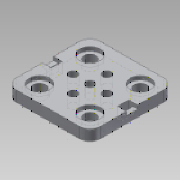
# Autodesk Inventor part: Micro V Plate
Saved by Autodesk Inventor 2013 SP2 (Build 170200200, 200)
## iProperties
IsCustomPart: 0
Created: 2013-06-20
Part Number: Micro V Plate
Material: Aluminum 6061
Document SubType Name: Modeling
Designer: Jon Hollander
Language: en-US
Size Designation: Micro V Plate
Categories: <MemberInstance><Categories><Category DisplayName="Other Parts" InternalName="5aa15e00-363f-49f2-933f-16f664388e3f" Mnemonic="OTHER"><Category DisplayName="Plates" InternalName="59c67330-93a2-418f-82cd-11a50f680607" Mnemonic="PLATES"/></Category><Category DisplayName="DataType" InternalName="23b78d0f-2648-40c6-8793-ca6db495c9e8" Mnemonic="DATATYPE"><CategoryParameter DisplayName="DisplayName" InternalName="05415f3d-3907-474b-a020-eb9d644f4cf3" Mnemonic="DISPLAYNAME"/><CategoryParameter DisplayName="InternalName" InternalName="cf1d0246-76d9-4b4a-8305-fa0409afb5c1" Mnemonic="INTERNALNAME"/><CategoryParameter DisplayName="Folder Name" InternalName="3f06958e-8713-4116-9be7-ed6184ecc97b" Mnemonic="FOLDERNAME"/><CategoryParameter DisplayName="Family Version" InternalName="914462f6-6e19-4b14-ba84-155b9680b1d0" Mnemonic="FAMILYREVISION"/><CategoryParameter DisplayName="ClipFormat" InternalName="bc51e27b-3422-4e78-93ef-cec197ddf230" Mnemonic="CLIPFORMAT"/><CategoryParameter DisplayName="IsMetric" InternalName="e2385c5b-1ea4-4823-96a8-8de651266ec3" Mnemonic="ISMETRIC"/><CategoryParameter DisplayName="Description" InternalName="13903e3d-64b1-4950-80da-f627842ea37f" Mnemonic="DESCRIPTION"/><CategoryParameter DisplayName="StdsOrg" InternalName="8f5914e1-4693-403f-8ab5-d37768198c9d" Mnemonic="STDSORG"/><CategoryParameter DisplayName="Standard" InternalName="0c0a119c-1e12-4c84-803f-101930972f5e" Mnemonic="STANDARD"/><CategoryParameter DisplayName="Manufacturer" InternalName="cd6c7a72-a28a-4e50-99a9-2c7f4e13e5ad" Mnemonic="MANUFACTURER"/><CategoryParameter DisplayName="Member Revision" InternalName="a65d44b9-392f-4f4f-857b-e4b3d54996fe" Mnemonic="MEMBERREVISION"/><CategoryParameter DisplayName="Standard Revision" InternalName="91d5a463-65c2-4fde-b823-3b7fea5e8e17" Mnemonic="STANDARDREVISION"/><CategoryParameter DisplayName="Revision Guid" InternalName="45a75005-10b1-4dfc-8d6d-dfe629f0b93c" Mnemonic="REVISIONGUID"/><CategoryParameter DisplayName="Designation" InternalName="2675968c-4ce5-49e0-a4f5-552d29089031" Mnemonic="DESIGNATION"/><CategoryParameter DisplayName="FileName" InternalName="8b46a4cc-9585-4fed-90c3-899f57e09a73" Mnemonic="FILENAME"/><CategoryParameter DisplayName="Default Row" InternalName="2af9ec52-faaa-4026-b378-f9fa4afca842" Mnemonic="DEFAULTROW"/><Category DisplayName="Part" InternalName="c0e0b642-3bcb-4cc8-9e80-f96d35c4afa4" Mnemonic="PART"><CategoryParameter DisplayName="Material" InternalName="818a152a-d3c3-49ca-80ee-df7d91421b8e" Mnemonic="MATERIAL"/><CategoryParameter DisplayName="Material Key" InternalName="5c9a8adb-dd2b-4535-b97f-0a94a95fe41f" Mnemonic="MATERIALKEY"/><CategoryParameter DisplayName="Part Number" InternalName="016b6077-bfbe-49bd-92c9-d8d59c39c941" Mnemonic="PARTNUMBER"/><CategoryParameter DisplayName="Stock Number" InternalName="4dba7c1c-e26c-444e-836c-b08b433409a8" Mnemonic="STOCKNUMBER"/></Category></Category></Categories><FamilyTemplate Id="Micro V Plate"><FamilyTemplateParameters><FamilyTemplateParameter ObjectType="kPartComponentDefinitionObject" ValueType="xs:string" Id="11" SubObjectId="Material"/><FamilyTemplateParameter ObjectType="kPropertyObject" ValueType="xs:string" Id="19" ObjectReferenceKey="{32853F0F-3444-11d1-9E93-0060B03C1CA6}" SubObjectId="5"/><FamilyTemplateParameter ObjectType="kPropertyObject" ValueType="xs:string" Id="20" ObjectReferenceKey="{32853F0F-3444-11d1-9E93-0060B03C1CA6}" SubObjectId="52"/></FamilyTemplateParameters></FamilyTemplate><CategoryParameterMap><ParamToTemplateMap><ParamToTemplate CategoryParameter="//CategoryParameter[@InternalName='cf1d0246-76d9-4b4a-8305-fa0409afb5c1']" ConstantValue="c0ed0d7d-6565-4805-8c82-f5f5bedef9ef"/><ParamToTemplate CategoryParameter="//CategoryParameter[@InternalName='45a75005-10b1-4dfc-8d6d-dfe629f0b93c']" ConstantValue="dbef3a4f-6e90-4593-8616-ded3e929c80e"/><ParamToTemplate CategoryParameter="//CategoryParameter[@InternalName='3f06958e-8713-4116-9be7-ed6184ecc97b']" ConstantValue="Micro V Plate"/><ParamToTemplate CategoryParameter="//CategoryParameter[@InternalName='8f5914e1-4693-403f-8ab5-d37768198c9d']" TemplateParameter="5"/><ParamToTemplate CategoryParameter="//CategoryParameter[@InternalName='0c0a119c-1e12-4c84-803f-101930972f5e']" TemplateParameter="6"/><ParamToTemplate CategoryParameter="//CategoryParameter[@InternalName='91d5a463-65c2-4fde-b823-3b7fea5e8e17']" TemplateParameter="7"/><ParamToTemplate CategoryParameter="//CategoryParameter[@InternalName='cd6c7a72-a28a-4e50-99a9-2c7f4e13e5ad']" TemplateParameter="8"/><ParamToTemplate CategoryParameter="//CategoryParameter[@InternalName='13903e3d-64b1-4950-80da-f627842ea37f']" TemplateParameter="10"/><ParamToTemplate CategoryParameter="//CategoryParameter[@InternalName='05415f3d-3907-474b-a020-eb9d644f4cf3']" ConstantValue="Micro V Plate"/><ParamToTemplate CategoryParameter="//CategoryParameter[@InternalName='914462f6-6e19-4b14-ba84-155b9680b1d0']" ConstantValue="11"/><ParamToTemplate CategoryParameter="//CategoryParameter[@InternalName='bc51e27b-3422-4e78-93ef-cec197ddf230']" ConstantValue="CF_INVENTOR.STDPARTS"/><ParamToTemplate CategoryParameter="//CategoryParameter[@InternalName='e2385c5b-1ea4-4823-96a8-8de651266ec3']" ConstantValue="true"/><ParamToTemplate CategoryParameter="//CategoryParameter[@InternalName='2af9ec52-faaa-4026-b378-f9fa4afca842']" ConstantValue="1"/><ParamToTemplate CategoryParameter="//CategoryParameter[@InternalName='8b46a4cc-9585-4fed-90c3-899f57e09a73']" ConstantValue="Micro V Plate"/><ParamToTemplate CategoryParameter="//CategoryParameter[@InternalName='a65d44b9-392f-4f4f-857b-e4b3d54996fe']" ConstantValue="f0f53da8-0783-4aef-9824-e74bb68f6a2c"/><ParamToTemplate CategoryParameter="//CategoryParameter[@InternalName='a65d44b9-392f-4f4f-857b-e4b3d54996fe']" ConstantValue="f0f53da8-0783-4aef-9824-e74bb68f6a2c"/><ParamToTemplate CategoryParameter="//CategoryParameter[@InternalName='2675968c-4ce5-49e0-a4f5-552d29089031']" TemplateParameter="20"/><ParamToTemplate CategoryParameter="//CategoryParameter[@InternalName='818a152a-d3c3-49ca-80ee-df7d91421b8e']" TemplateParameter="11"/><ParamToTemplate CategoryParameter="//CategoryParameter[@InternalName='016b6077-bfbe-49bd-92c9-d8d59c39c941']" TemplateParameter="19"/></ParamToTemplateMap></CategoryParameterMap></MemberInstance>
Mass: 35.4792 g
Surface Area: 69.5498 cm^2
Volume: 13.092 cm^3
Density: 2.71 g/cm^3
Author: Jon Hollander
Autodesk Inventor part; units mm, degrees
ref_plane "Work Plane1" through (0, -18.83, 0) normal (-1, 0, 0) x (0, 0, 1)
ref_plane "YZ Plane" through (0, 0, 0) normal (1, 0, 0) x (0, 1, 0)
ref_plane "XZ Plane" through (0, 0, 0) normal (0, 1, 0) x (-1, 0, 0)
sketch "Sketch1" plane through (0, 0, 0) normal (0, 0, 1) x (1, 0, 0)
  line L0 (-25, -25) -> (25, -25)
  line L1 (25, -25) -> (25, 25)
  line L2 (25, 25) -> (-25, 25)
  line L3 (-25, 25) -> (-25, -25)
  line L4 (-25, -25) -> (25, 25) construction
  line L5 (25, -25) -> (-25, 25) construction
  point P0 (0, 0)
  dimension "Width" = 50
  dimension "Height" = 50
  constraints: 12 end point, 2 midpoint, 2 parallel, 1 horizontal, 1 perpendicular
  measures "Width" distance of L2.end L1.end
  measures "Height" distance of L0.end L1.end
extrude "Extrusion1" add sketch "Sketch1" along normal blind 6.35
sketch "Sketch2" plane through (0, 0, 6.35) normal (0, 0, 1) x (1, 0, 0)
  line L0 (-25, -25) -> (25, -25) projected
  line L1 (25, -25) -> (25, 25) projected
  line L2 (25, 25) -> (-25, 25) projected
  line L3 (-25, 25) -> (-25, -25) projected
  line L4 (0, 25) -> (0, -25) construction
  line L5 (-25, 0) -> (25, 0) construction
  point P0 (0, 0)
  point P1 (0, 0)
  point P2 (-10, 0)
  point P3 (0, 10)
  point P4 (0, -10)
  point P5 (10, 0)
  dimension "d4" = 10
  dimension "d5" = 10
  dimension "d6" = 10
  dimension "d7" = 10
  constraints: 4 end point, 4 midpoint, 4 point on line, 1 coincident
  measures "d4" distance of point (0, 0) point (-10, 0)
  measures "d5" distance of point (10, 0) point (0, 0)
  measures "d6" distance of point (0, 10) point (0, 0)
  measures "d7" distance of point (0, -10) point (0, 0)
hole "Hole1" at (0, 0, 6.35) at (-10, 0, 6.35) at (0, 10, 6.35) at (0, -10, 6.35) at (10, 0, 6.35) direction (0, 0, -1) diameter 5.02 end through all
sketch "Sketch3" plane through (0, 0, 6.35) normal (0, 0, 1) x (1, 0, 0)
  line L0 (-25, -25) -> (25, -25) projected
  line L1 (25, -25) -> (25, 25) projected
  line L2 (25, 25) -> (-25, 25) projected
  line L3 (-25, 25) -> (-25, -25) projected
  line L4 (0, 25) -> (0, -25) construction
  line L5 (25, 0) -> (-25, 0) construction
  line L6 (15, 25) -> (15, -25) construction
  line L7 (-25, -15) -> (25, -15) construction
  point P0 (15, 15)
  point P1 (-15, 15)
  dimension "d15" = 15
  dimension "d16" = 15
  constraints: 8 end point, 4 midpoint, 4 point on line, 2 perpendicular
  measures "d15" distance between parallel lines of L6 L4
  measures "d16" distance between parallel lines of L5 L7
hole "Hole2" at (-15, 15, 6.35) at (15, 15, 6.35) direction (0, 0, -1) diameter 7.14 end through all counterbore diameter 12 counterbore depth 2.18
sketch "Sketch6" plane through (0, 0, 6.35) normal (0, 0, 1) x (1, 0, 0)
  circle A0 centre (-15, 15) radius 6 projected
  circle A1 centre (15, 15) radius 6 projected
  circle A2 centre (0, -10) radius 2.51 projected
  circle A3 centre (-10, 0) radius 2.51 projected
  circle A4 centre (0, 0) radius 2.51 projected
  circle A5 centre (0, 10) radius 2.51 projected
  circle A6 centre (10, 0) radius 2.51 projected
  line L0 (-25, -25) -> (25, -25) projected
  line L1 (25, -25) -> (25, 25) projected
  line L2 (25, 25) -> (-25, 25) projected
  line L3 (-25, 25) -> (-25, -25) projected
sketch "Sketch7" plane through (0, 0, 6.35) normal (0, 0, 1) x (1, 0, 0)
  circle A0 centre (-15, 15) radius 6 projected
  circle A1 centre (15, 15) radius 6 projected
  line L0 (-25, -25) -> (25, -25) projected
  line L1 (25, -25) -> (25, 25) projected
  line L2 (-25, 25) -> (-25, -25) projected
  line L3 (15, 15) -> (15, -25) construction
  line L4 (25, -16.9) -> (-25, -16.9) construction
  line L5 (-15, 15) -> (-15, -16.9) construction
  point P0 (15, -16.9)
  dimension "d35" = 31.9
  constraints: 6 end point, 6 point on line, 3 perpendicular, 1 coincident
  measures "d35" distance from line of L4 L3.start
hole "Hole3" at (-15, -16.9, 6.35) at (15, -16.9, 6.35) direction (0, 0, -1) diameter 5 end through all counterbore diameter 10.1 counterbore depth 2
sketch "Sketch4" plane through (0, 0, 6.35) normal (0, 0, 1) x (1, 0, 0)
  line L0 (25, -18.83) -> (25, 18.83) projected
  line L1 (-25, 18.83) -> (-25, -18.83) projected
  line L2 (-25, 0) -> (25, 0) construction
  line L3 (-22.25, 3.35) -> (-19.75, 3.35)
  line L4 (-19.75, 3.35) -> (-19.75, -3.35)
  line L5 (-19.75, -3.35) -> (-22.25, -3.35)
  line L6 (-22.25, -3.35) -> (-22.25, 3.35)
  line L7 (-22.25, 3.35) -> (-19.75, -3.35) construction
  line L8 (-19.75, 3.35) -> (-22.25, -3.35) construction
  point P0 (-21, 0)
  dimension "d25" = 2.5
  dimension "d27" = 5.25
  dimension "d28" = 6.7
  constraints: 14 end point, 4 midpoint, 2 parallel, 1 horizontal, 1 perpendicular, 1 point on line
  measures "d25" distance of L3.start L3.end
  measures "d27" distance between parallel lines of L1 L4
  measures "d28" distance of L3.end L4.end
sketch "Sketch5" plane through (-25, -18.83, 0) normal (-1, 0, 0) x (0, 0, 1)
  line L0 (6.35, 37.66) -> (6.35, 0) projected
  line L1 (0, 15.48) -> (0, 22.18) projected
  line L2 (6.35, 22.18) -> (0, 22.18) projected
  line L3 (6.35, 15.48) -> (0, 15.48) projected
  line L4 (6.35, 22.18) -> (4.17, 22.18)
  line L5 (4.17, 22.18) -> (4.17, 15.48)
  line L6 (4.17, 15.48) -> (6.35, 15.48)
  line L7 (6.35, 15.48) -> (6.35, 22.18)
  point P0 (0, 18.83)
  dimension "d31" = 2.18
  constraints: 8 end point, 2 parallel, 1 horizontal, 1 perpendicular, 1 point on line
  measures "d31" distance between parallel lines of L7 L5
body "Solid1"
